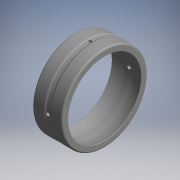
# Autodesk Inventor part: 22205/20 E_or
Saved by Autodesk Inventor 2017.3 (Build 213256000, 256)
## iProperties
Part Number: 22205/20 E_or
Material: Generic
Catalog Web Link: www.cadenas.de
Description: BS2_001-Spherical roller bearings
Vendor: SKF
Document SubType Name: Modeling
Designer: partserver
Manufacturer: SKF
Mass: 7.49151 g
Surface Area: 66.5855 cm^2
Volume: 7.49151 cm^3
Density: 1 g/cm^3
Appearance: PSOLRGB-175-175-175
Category: PARTsolutions
Company: SKF
Title: 22205/20 E_or
Author: Cadenas PARTsolutions
Comments: Spherical roller bearings
PSOL_IDENT_0: {$CADENAS_DATA\23d-libs\skf\bearings_units_and_housings\roller_bearings\spherical_roller_bearings\pa
PSOL_IDENT_1: rts\bs2_001_or.prj},171 {VTYP=3D},{NB=22205/20 E_or},{LINA=22205/20 E_or},{NN=BS2_001},{DATE=23.12.2
PSOL_IDENT_2: 020 11:58:30},{GEOMDATE=24.11.2020 12:50:21},{VERSION=},{LINEID=460970},{WBVAR=},{WBNUMERIC=}  {NB=2
PSOL_IDENT_3: 2205/20 E_or},{LINA=22205/20 E_or},{KT=DUMMY},{DESIGNATION=22205/20 E},{VARIANT=CE1W33},{DESIGNX=Cyl
PSOL_IDENT_4: indrical bore},{SEAL=No seals},{SALG=NO},{BORE=20.000},{DD=20.000},{DD1=MIN},{D=52.000},{B=18.000},{
PSOL_IDENT_5: DD2=31.300},{DD3=MIN},{D1=44.200},{B1=MIN},{B2=MIN},{B4=MIN},{B5=MIN},{BB=3.700},{K=2.000},{R12=1.00
PSOL_IDENT_6: 0},{G=},{G1=MIN},{TB=MIN},{ALPHA=12.8333},{R34=MIN},{PITCH=39.459},{DW=7.130},{LW=6.600},{DDAMIN=25.
PSOL_IDENT_7: 600},{DDAMAX=MIN},{DBMIN=MIN},{DAMAX=46.400},{BAMIN=MIN},{RAMAX=1.000},{LOAD1=49.900},{LOAD2=44.000}
PSOL_IDENT_8: ,{LOAD3=4.750},{SPEED1=13000},{SPEED2=17000},{PRA=},{PLA=},{Z=15.000},{II=2.000},{MASS=0.280},{MASS2=
PSOL_IDENT_9: MIN},{SLEEVE=},{POPULAR=},{BEARING=22205/20 E},{PPATH=parts/bs2_001_asmtpl.prj},{RAMAXX=1},{EE=0.35}
PSOL_IDENT_10: ,{Y0=1.8},{R12X=1},{Y2=2.9},{ALPHAX=12.83333},{Y1=1.9},{DD1X=},{B1X=},{SLEEVEX=},{ALPHAXX=},{B2X=},{
PSOL_IDENT_11: SUPRESSED=},{BBALG=3.700},{KALG=2.000},{Y=0.000}
NB: 22205/20 E_or
NN: BS2_001
NT: Spherical roller bearings
NBSYN: $DESIGNATION._or
LINA: 22205/20 E_or
CATALOG: SKF
DESIGNATION: 22205/20 E
VARIANT: CE1W33
DESIGNX: Cylindrical bore
SEAL: No seals
BORE: 20
DD: 20
DD1: 0
D: 52
B: 18
DD2: 31.3
DD3: 0
D1: 44.2
B1: 0
B2: 0
B4: 0
B5: 0
BB: 3.7
K: 2
R12: 1
G1: 0
TB: 0
ALPHA: 12.8333
R34: 0
PITCH: 39.459
DW: 7.13
LW: 6.6
DDAMIN: 25.6
DDAMAX: 0
DBMIN: 0
DAMAX: 46.4
BAMIN: 0
RAMAX: 1
LOAD1: 49.9
LOAD2: 44
LOAD3: 4.75
SPEED1: 13000
SPEED2: 17000
Z: 15
II: 2
MASS: 0.28
MASS2: 0
BEARING: 22205/20 E
PPATH: parts/bs2_001_asmtpl.prj
RAMAXX: 1
EE: 0.35
Y0: 1.8
R12X: 1
Y2: 2.9
ALPHAX: 12.83333
Y1: 1.9
Y: 0
SUPPLIER: SKF
ARTICLENO: 22205/20 E_or
BOMINFO: 22205/20 E_or
CREATOR: CADENAS GmbH
Autodesk Inventor part; units mm, degrees
sketch "Sketch_5" plane through (0, 0, 0) normal (0, 0, 1) x (1, 0, 0)
  line L0 (18, 0) -> (-18, 0)
  arc A0 (0, 22.3978) -> (0.3417, 22.1652) centre (0.25, 22.3978) ccw
  arc A1 (6.5373, 23.669) -> (0.3417, 22.1652) centre (8.8822, 0.4928) ccw
  arc A2 (11.4627, 23.669) -> (6.5373, 23.669) centre (9, -326.3223) ccw
  arc A3 (17.6583, 22.1652) -> (11.4627, 23.669) centre (9.1178, 0.4928) ccw
  arc A4 (17.6583, 22.1652) -> (18, 22.3978) centre (17.75, 22.3978) ccw
  line L1 (18, 22.3978) -> (18, 25)
  arc A5 (18, 25) -> (17, 26) centre (17, 25) ccw
  line L2 (17, 26) -> (10.85, 26)
  line L3 (10.85, 26) -> (10, 25.575)
  line L4 (10, 25.575) -> (8, 25.575)
  line L5 (8, 25.575) -> (7.15, 26)
  line L6 (7.15, 26) -> (1, 26)
  arc A6 (1, 26) -> (0, 25) centre (1, 25) ccw
  line L7 (0, 25) -> (0, 22.3978)
  constraints: 16 end point, 14 point on circle, 7 centre point
revolve "Revolution1" add sketch "Sketch_5" angle 360 about axis through (18, 0, 0) along (1, 0, 0)
sketch "Sketch_2" plane through (0, 0, 0) normal (0, 0, 1) x (1, 0, 0)
  line L0 (9, -26) -> (9, -22.1)
  line L1 (9, -22.1) -> (10, -22.1)
  line L2 (10, -22.1) -> (10, -26)
  line L3 (10, -26) -> (9, -26)
  line L4 (9, -26) -> (9, -22.1)
  constraints: 10 end point
revolve "Revolution2" cut sketch "Sketch_2" angle 360 about axis through (9, -26, 0) along (0, -1, 0)
sketch "Sketch_9" plane through (0, 0, 0) normal (0, 1, 0) x (-1, 0, 0)
  line L0 (-9, -22.1) -> (-9, -26)
  line L1 (-9, -26) -> (-10, -26)
  line L2 (-10, -26) -> (-10, -22.1)
  line L3 (-10, -22.1) -> (-9, -22.1)
  line L4 (-9, -22.1) -> (-9, -26)
  constraints: 10 end point
revolve "Revolution3" cut sketch "Sketch_9" angle 360 about axis through (9, 0, -22.1) along (0, 0, 1)
sketch "Sketch_10" plane through (0, 0, 0) normal (0, 0, 1) x (1, 0, 0)
  line L0 (9, 22.1) -> (9, 26)
  line L1 (9, 26) -> (10, 26)
  line L2 (10, 26) -> (10, 22.1)
  line L3 (10, 22.1) -> (9, 22.1)
  line L4 (9, 22.1) -> (9, 26)
  constraints: 10 end point
revolve "Revolution4" cut sketch "Sketch_10" angle 360 about axis through (9, 22.1, 0) along (0, -1, 0)
ref_plane "NO_GEO_XY" through (0, 0, 0) normal (1, 0, 0) x (0, 0, -1)
ref_plane "NO_GEO_YZ" through (0, 0, 0) normal (0, 0, -1) x (0, 1, 0)
ref_plane "NO_GEO_ZX" through (0, 0, 0) normal (0, 1, 0) x (1, 0, 0)
ref_plane "or_XY" through (0, 0, 0) normal (0, 0, 1) x (1, 0, 0)
ref_plane "or_YZ" through (0, 0, 0) normal (1, 0, 0) x (0, 1, 0)
ref_plane "or_ZX" through (0, 0, 0) normal (0, 1, 0) x (0, 0, 1)
body "Solid1"
